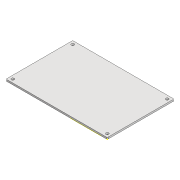
# Autodesk Inventor part: Base
Saved by Autodesk Inventor 2020 (Build 240168000, 168)
## iProperties
Created: 2022-07-16
Part Number: Base
Material: Genérico
Document SubType Name: Modeling
Designer: gabri
Density: 1 g/cm^3
Appearance: Padrão
Author: gabri
Autodesk Inventor part; units mm, degrees
ref_plane "YZ Plane" through (0, 0, 0) normal (1, 0, 0) x (0, 1, 0)
ref_plane "XZ Plane" through (0, 0, 0) normal (0, 1, 0) x (-1, 0, 0)
ref_plane "XY Plane" through (0, 0, 0) normal (0, 0, 1) x (1, 0, 0)
sketch "Esboço1" plane through (0, 0, 0) normal (0, 1, 0) x (-1, 0, 0)
  line L0 (0, 0) -> (252, 0)
  line L1 (252, 0) -> (252, -158)
  line L2 (252, -158) -> (0, -158)
  line L3 (0, -158) -> (0, 0)
  dimension "d0" = 252
  dimension "d1" = 158
  constraints: 8 end point, 2 parallel, 1 horizontal, 1 perpendicular
  measures "d0" distance of L1.end L2.end
  measures "d1" distance of L0.end L1.end
extrude "Extrusão1" add sketch "Esboço1" along normal blind 4
fillet "Arredondamento1" radius 2 4 edges at (0, 2, 0) (0, 2, -158) (-252, 2, 0) (-252, 2, -158)
sketch "Esboço2" plane through (0, 4, 0) normal (0, 1, 0) x (1, 0, 0)
  circle A0 centre (-244, 150) radius 3.35
  circle A1 centre (-244, 8) radius 3.35
  circle A2 centre (-8, 150) radius 3.35
  circle A3 centre (-8, 8) radius 3.35
  line L0 (-252, 156) -> (-252, 2) projected
  line L1 (-2, 158) -> (-250, 158) projected
  line L2 (-250, 0) -> (-2, 0) projected
  line L3 (0, 2) -> (0, 156) projected
  point P0 (0, 0)
  dimension "d5" = 6.7
  dimension "d6" = 6.7
  dimension "d7" = 6.7
  dimension "d8" = 6.7
  dimension "d9" = 8
  dimension "d10" = 8
  dimension "d11" = 8
  dimension "d12" = 8
  dimension "d13" = 8
  dimension "d14" = 8
  dimension "d15" = 8
  dimension "d16" = 8
  constraints: 4 centre point
  measures "d5" diameter of A1
  measures "d6" diameter of A2
  measures "d7" diameter of A3
  measures "d8" diameter of A0
  measures "d9" distance from line of L0 A0.centre
  measures "d10" distance from line of L1 A0.centre
  measures "d11" distance from line of L2 A1.centre
  measures "d12" distance from line of L0 A1.centre
  measures "d13" distance from line of L3 A3.centre
  measures "d14" distance from line of L2 A3.centre
  measures "d15" distance from line of L3 A2.centre
  measures "d16" distance from line of L1 A2.centre
extrude "Extrusão2" cut sketch "Esboço2" against normal blind 10
sketch "Esboço3" plane through (0, 0, 0) normal (0, -1, 0) x (1, 0, 0)
  line L0 (-14.2, -140.75) -> (-87.5029, -140.75) projected
  arc A0 (-89.0029, -139.25) -> (-87.5029, -140.75) centre (-87.5029, -139.25) ccw projected
  line L1 (-89.0029, -130.5) -> (-89.0029, -139.25) projected
  line L2 (-89.0029, -130.5) -> (-89.0029, -10.5) projected
  line L3 (-89.0029, -1.75) -> (-89.0029, -10.5) projected
  arc A1 (-87.5029, -0.25) -> (-89.0029, -1.75) centre (-87.5029, -1.75) ccw projected
  line L4 (-87.5029, -0.25) -> (-14.2, -0.25) projected
  line L5 (-14.2, -140.75) -> (-14.2, -0.25) projected
  circle A2 centre (-31, -21) radius 2 projected
  circle A3 centre (-31, -21) radius 4 projected
  circle A4 centre (-41, -31) radius 2 projected
  circle A5 centre (-31, -21) radius 2 projected
  circle A6 centre (-31, -121) radius 4.5 projected
  circle A7 centre (-82, -111) radius 2 projected
  circle A8 centre (-41, -111) radius 2 projected
  circle A9 centre (-72, -121) radius 2 projected
  circle A10 centre (-72, -121) radius 4.5 projected
  circle A11 centre (-41, -31) radius 2 projected
  circle A12 centre (-82, -31) radius 2 projected
  circle A13 centre (-72, -21) radius 2 projected
  circle A14 centre (-72, -21) radius 4.5 projected
  point P0 (0, 0)
extrude "Extrusão3" cut sketch "Esboço3" against normal blind 10 contours A4 | A7 | A8 | A12
sketch "Esboço4" plane through (0, 4, 0) normal (0, 1, 0) x (1, 0, 0)
  circle A0 centre (-216, 148) radius 2 projected
  circle A1 centre (-108, 137) radius 2 projected
  circle A2 centre (-119, 149) radius 2 projected
  circle A3 centre (-228, 137) radius 2 projected
  circle A4 centre (-227, 21) radius 2 projected
  circle A5 centre (-216, 9) radius 2 projected
  circle A6 centre (-108, 21) radius 2 projected
  circle A7 centre (-119, 9) radius 2 projected
  point P0 (0, 0)
  point P1 (-122.4, 150.963)
  constraints: 1 other
extrude "Extrusão4" cut sketch "Esboço4" against normal blind 10
equation "\"d8\" = d6"
equation "\"d10\" = d12"
equation "\"d11\" = d10"
equation "\"d12\" = d9"
equation "\"d13\" = d12"
equation "\"d14\" = d13"
equation "\"d15\" = d13"
equation "\"d16\" = d15"
